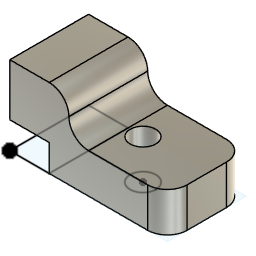
Backlight_Clamp_Right (Autodesk Fusion 360 design; units mm, degrees)
part number: 2025-07-08-11-33-51-161
Autodesk Fusion 360 part; units mm, degrees
sketch "Sketch1" plane through (0, 0, 0) normal (0, 0, 1) x (1, 0, 0)
  line L0 (0, 0) -> (40, 0)
  line L1 (40, 0) -> (40, 20)
  line L2 (40, 20) -> (0, 20)
  line L3 (0, 20) -> (0, 0)
  dimension "d1" = 40
  dimension "d2" = 20
  constraint horizontal L0
  constraint vertical L1
  constraint horizontal L2
  constraint vertical L3
  constraint coincident L0.start L3.end
  measures "d1" distance of L0.start L0.end
  measures "d2" distance of L0.start L2.end
extrude "Extrude1" add sketch "Sketch1" along normal blind 20
sketch "Sketch2" plane through (0, 0, 0) normal (0, 0, -1) x (1, 0, 0)
  line L0 (0, 0) -> (0, -20)
  line L1 (0, -20) -> (40, -20)
  line L2 (40, -20) -> (40, 0)
  line L3 (40, 0) -> (0, 0)
  line L4 (0, 0) -> (10, 0)
  line L5 (10, 0) -> (10, -20)
  line L6 (10, -20) -> (0, -20)
  line L7 (0, -20) -> (0, 0)
  line L8 (10, -10) -> (23.8, -10)
  circle A0 centre (23.8, -10) radius 3.25
  dimension "d5" = 10
  dimension "d6" = 20
  dimension "d7" = 13.8
  dimension "d8" = 6.5
  constraint horizontal L4
  constraint vertical L5
  constraint horizontal L6
  constraint vertical L7
  constraint coincident L0.start L3.end
  constraint horizontal L8
  constraint midpoint L5 L8.start
  constraint coincident L8.end A0.centre
  measures "d5" distance of L0.start L4.end
  measures "d6" distance of L0.start L0.end
  measures "d7" distance of L8.start L8.end
  measures "d8" diameter of A0
extrude "Extrude2" cut sketch "Sketch2" against normal blind 7.8 contours L0 L1 L3 L4 L5 L6 L7 | A0
extrude "Extrude3" cut 1 faces at (24.5115, 8.6722, 7.8) along direction (0, 0, 1) blind 210
sketch "Sketch3" plane through (0, 0, 20) normal (0, 0, 1) x (-1, 0, 0)
  circle A0 centre (-23.8, -10) radius 3.25
  line L0 (0, -20) -> (0, 0)
  line L1 (0, 0) -> (-40, 0)
  line L2 (-40, 0) -> (-40, -20)
  line L3 (-40, -20) -> (0, -20)
  line L4 (-40, -20) -> (-15, -20)
  line L5 (-15, -20) -> (-15, 0)
  line L6 (-15, 0) -> (-40, 0)
  line L7 (-40, 0) -> (-40, -20)
  dimension "d13" = 25
  dimension "d14" = 20
  constraint horizontal L4
  constraint vertical L5
  constraint horizontal L6
  constraint vertical L7
  constraint coincident L2.end L3.start
  measures "d13" distance of L2.end L4.end
  measures "d14" distance of L2.end L1.end
extrude "Extrude4" cut sketch "Sketch3" against normal blind 10 contours L1 L2 L3 L4 L5 L6 L7
fillet "Fillet1" radius 5 2 edges at (15, 10, 10) (15, 10, 20)
fillet "Fillet2" radius 5 2 edges at (40, 0, 5) (40, 20, 5)
sketch "Sketch4" plane through (0, 0, 0) normal (0, 1, 0) x (1, 0, 0)
extrude "Extrude5" cut 1 faces at (10, 6.6667, 2.6) along direction (1, 0, 0) blind 0.5
extrude "Extrude6" add 1 faces at (10.5, 6.6667, 2.6) along direction (-1, 0, 0) blind 0.5
sketch "Sketch5" plane through (0, 0, 20) normal (0, 0, 1) x (-1, 0, 0)
  line L0 (-10, 0) -> (-10, -20)
  line L1 (-10, -20) -> (0, -20)
  line L2 (0, -20) -> (0, 0)
  line L3 (0, 0) -> (-10, 0)
sketch "Sketch6" plane through (0, 0, 0) normal (0, -1, 0) x (1, 0, 0)
  line L0 (10, 0) -> (35, 0)
  line L1 (35, 0) -> (35, 10)
  line L2 (35, 10) -> (20, 10)
  arc A0 (15, 15) -> (20, 10) centre (20, 15) ccw
  arc A1 (15, 15) -> (10, 20) centre (10, 15) ccw
  line L3 (10, 20) -> (0, 20)
  line L4 (0, 20) -> (0, 7.8)
  line L5 (0, 7.8) -> (10, 7.8)
  line L6 (10, 7.8) -> (10, 0)
sketch "Sketch7" plane through (0, 0, 0) normal (0, -1, 0) x (1, 0, 0)
sketch "Sketch8" plane through (0, 0, 10) normal (0, 0, 1) x (-1, 0, 0)
  arc A0 (-40, -15) -> (-35, -20) centre (-35, -15) ccw
  line L0 (-35, -20) -> (-20, -20)
  line L1 (-20, -20) -> (-20, 0)
  line L2 (-20, 0) -> (-35, 0)
  arc A1 (-35, 0) -> (-40, -5) centre (-35, -5) ccw
  line L3 (-40, -5) -> (-40, -15)
  circle A2 centre (-23.8, -10) radius 3.25
extrude "Extrude7" add 1 faces at (3.3333, 6.6667, 7.8) along direction (0, 0, -1) blind 1
